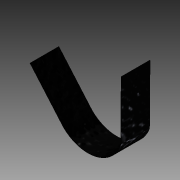
# Autodesk Inventor part: Sheild
Saved by Autodesk Inventor 2013 (Build 170138000, 138)
## iProperties
Created: 2013-06-28
Part Number: Sheild
Material: Generic
Document SubType Name: Modeling
Designer: mvarma
Density: 1 g/cm^3
Author: mvarma
Autodesk Inventor part; units mm, degrees
ref_plane "YZ Plane" through (0, 0, 0) normal (1, 0, 0) x (0, 1, 0)
ref_plane "XZ Plane" through (0, 0, 0) normal (0, 1, 0) x (-1, 0, 0)
ref_plane "XY Plane" through (0, 0, 0) normal (0, 0, 1) x (1, 0, 0)
sketch "Sketch1" plane through (0, 0, 0) normal (0, 0, 1) x (1, 0, 0)
  arc A0 (66.7702, 112.6298) -> (73.6141, 138.1061) centre (52.5264, 130.1136) ccw construction
  line L0 (63.1006, 61.9455) -> (112.0149, 5.088)
  arc A1 (66.7702, 112.6298) -> (63.1006, 61.9455) centre (88.8254, 85.558) ccw construction
  arc A2 (138.8831, 162.8706) -> (162.2319, 146.2144) centre (163.0457, 172.0484) ccw construction
  arc A3 (172.0845, 144.47) -> (162.2319, 146.2144) centre (161.1324, 111.3067) ccw construction
  line L1 (196.0564, 111.0477) -> (195.4211, 25.3647)
  arc A4 (112.0149, 5.088) -> (112.3757, 4.7043) centre (116.5302, 8.9726) ccw
  arc A5 (112.3757, 4.7043) -> (195.1395, 23.7862) centre (147.6111, 40.9044) ccw
  arc A6 (195.1395, 23.7862) -> (195.4211, 25.3647) centre (190.6588, 25.4) ccw
  arc A7 (196.0564, 111.0477) -> (172.0845, 144.47) centre (161.1324, 111.3067) ccw construction
  arc A8 (138.8831, 162.8706) -> (73.6141, 138.1061) centre (105.8063, 151.6542) ccw construction
  line L2 (111.4132, 4.5704) -> (62.5072, 61.4182)
  arc A9 (66.2689, 113.2452) -> (62.5072, 61.4182) centre (88.8254, 85.558) ccw construction
  arc A10 (66.2689, 113.2452) -> (72.8769, 137.8116) centre (52.5264, 130.1136) ccw construction
  arc A11 (139.6302, 163.1392) -> (72.8769, 137.8116) centre (105.8063, 151.6542) ccw construction
  arc A12 (139.6302, 163.1392) -> (162.2569, 147.0077) centre (163.0457, 172.0484) ccw construction
  arc A13 (172.3334, 145.2237) -> (162.2569, 147.0077) centre (161.1324, 111.3067) ccw construction
  arc A14 (196.8501, 111.0418) -> (172.3334, 145.2237) centre (161.1324, 111.3067) ccw construction
  line L3 (196.8501, 111.0418) -> (196.2148, 25.3588)
  arc A15 (195.8863, 23.5172) -> (196.2148, 25.3588) centre (190.6588, 25.4) ccw
  arc A16 (111.8221, 4.1355) -> (195.8863, 23.5172) centre (147.6111, 40.9044) ccw
  arc A17 (111.4132, 4.5704) -> (111.8221, 4.1355) centre (116.5302, 8.9726) ccw
  line L4 (196.0564, 111.0477) -> (196.8501, 111.0418)
  line L5 (63.1006, 61.9455) -> (62.5072, 61.4182)
  point P0 (0, 0)
  point P1 (93.7791, 184.445)
  point P2 (71.0776, 147.9379)
  point P3 (60.2024, 105.5589)
  point P4 (195.6522, 56.526)
  point P5 (134.0244, 172.2363)
  dimension "d0" = 0.7937
  constraints: 40 point on circle, 18 centre point, 12 end point, 2 tangent, 1 perpendicular, 1 point on line, 45 other
  measures "d0" distance between parallel lines of L0 L2
extrude "Extrusion1" add sketch "Sketch1" along normal blind 42.164
body "Solid1"
